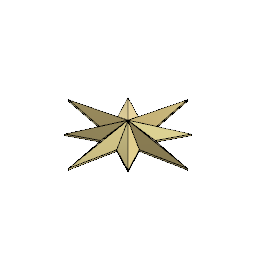
Star (Autodesk Fusion 360 design; units mm, degrees)
Autodesk Fusion 360 part; units mm, degrees
sketch "Outline" plane through (0, 0, 0) normal (0, 0, 1) x (1, 0, 0)
  line L0 (0, 0) -> (82.1329, 34.0206) construction
  line L1 (0, 0) -> (34.0206, 82.1329) construction
  line L2 (0, 0) -> (82.1329, -34.0206) construction
  line L3 (0, 0) -> (34.0206, -82.1329) construction
  line L4 (0, 0) -> (-82.1329, 34.0206) construction
  line L5 (0, 0) -> (-34.0206, -82.1329) construction
  line L6 (0, 0) -> (-82.1329, -34.0206) construction
  line L7 (0, 0) -> (-34.0206, 82.1329)
  line L8 (82.1329, 34.0206) -> (134.7038, 134.7038)
  line L9 (134.7038, 134.7038) -> (34.0206, 82.1329)
  line L10 (254, 0) -> (82.1329, 34.0206)
  line L11 (82.1329, -34.0206) -> (254, 0)
  line L12 (134.7038, -134.7038) -> (82.1329, -34.0206)
  line L13 (34.0206, -82.1329) -> (134.7038, -134.7038)
  line L14 (34.0206, 82.1329) -> (0, 254)
  line L15 (0, 254) -> (-34.0206, 82.1329)
  line L16 (-34.0206, 82.1329) -> (-134.7268, 134.6809)
  line L17 (-134.7268, 134.6809) -> (-82.1329, 34.0206)
  line L18 (-82.1329, 34.0206) -> (-254, 0)
  line L19 (-254, 0) -> (-82.1329, -34.0206)
  line L20 (-82.1329, -34.0206) -> (-134.7038, -134.7038)
  line L21 (-134.7038, -134.7038) -> (-34.0206, -82.1329)
  line L22 (-34.0206, -82.1329) -> (0, -254)
  line L23 (0, -254) -> (34.0206, -82.1329)
  line L24 (-134.7268, 134.6809) -> (0, 0) construction
  line L25 (0, 0) -> (134.7038, -134.7038) construction
  line L26 (0, 0) -> (0, 254) construction
  line L27 (0, 0) -> (134.7038, 134.7038) construction
  line L28 (0, 0) -> (0, -254) construction
  line L29 (-134.7038, -134.7038) -> (0, 0) construction
  line L30 (0, 0) -> (-254, 0) construction
  line L31 (0, 0) -> (254, 0) construction
  circle A0 centre (0, 0) radius 11.95 construction
  circle A1 centre (8.2884, 8.6084) radius 2.1
  circle A2 centre (-8.6084, 8.2884) radius 2.1
  circle A3 centre (-8.2884, -8.6084) radius 2.1
  circle A4 centre (8.6084, -8.2884) radius 2.1
  circle A5 centre (0, 0) radius 16.2
  line L32 (4.3489, 7.4725) -> (7.3024, 4.6287)
  line L33 (7.3024, 4.6287) -> (11.2419, 5.7647)
  line L34 (11.2419, 5.7647) -> (12.2279, 9.7444)
  line L35 (12.2279, 9.7444) -> (9.2744, 12.5881)
  line L36 (9.2744, 12.5881) -> (5.3349, 11.4521)
  line L37 (5.3349, 11.4521) -> (4.3489, 7.4725)
  line L38 (-7.4725, 4.3489) -> (-4.6287, 7.3024)
  line L39 (-4.6287, 7.3024) -> (-5.7647, 11.2419)
  line L40 (-5.7647, 11.2419) -> (-9.7444, 12.2279)
  line L41 (-9.7444, 12.2279) -> (-12.5881, 9.2744)
  line L42 (-12.5881, 9.2744) -> (-11.4521, 5.3349)
  line L43 (-11.4521, 5.3349) -> (-7.4725, 4.3489)
  line L44 (-11.2419, -5.7647) -> (-12.2279, -9.7444)
  line L45 (-12.2279, -9.7444) -> (-9.2744, -12.5881)
  line L46 (-9.2744, -12.5881) -> (-5.3349, -11.4521)
  line L47 (-5.3349, -11.4521) -> (-4.3489, -7.4725)
  line L48 (-4.3489, -7.4725) -> (-7.3024, -4.6287)
  line L49 (-7.3024, -4.6287) -> (-11.2419, -5.7647)
  line L50 (11.4521, -5.3349) -> (7.4725, -4.3489)
  line L51 (7.4725, -4.3489) -> (4.6287, -7.3024)
  line L52 (4.6287, -7.3024) -> (5.7647, -11.2419)
  line L53 (5.7647, -11.2419) -> (9.7444, -12.2279)
  line L54 (9.7444, -12.2279) -> (12.5881, -9.2744)
  line L55 (12.5881, -9.2744) -> (11.4521, -5.3349)
  line L56 (-82.1329, 34.0206) -> (-34.0206, 82.1329)
  line L57 (34.0206, 82.1329) -> (-34.0206, 82.1329)
  line L58 (34.0206, 82.1329) -> (82.1329, 34.0206)
  line L59 (82.1329, 34.0206) -> (82.1329, -34.0206)
  line L60 (82.1329, -34.0206) -> (34.0206, -82.1329)
  line L61 (34.0206, -82.1329) -> (-34.0206, -82.1329)
  line L62 (-34.0206, -82.1329) -> (-82.1329, -34.0206)
  line L63 (-82.1329, -34.0206) -> (-82.1329, 34.0206)
  line L64 (4.6287, -7.3024) -> (0, 0) construction
  line L65 (7.4725, -4.3489) -> (0, 0) construction
  line L66 (0, 0) -> (7.3024, 4.6287) construction
  line L67 (4.3489, 7.4725) -> (0, 0) construction
  circle A6 centre (0, 0) radius 25.4
  circle A7 centre (0, 0) radius 25.146
  circle A8 centre (0, 0) radius 4.1
  line L68 (-4.3489, -7.4725) -> (0, 0) construction
  line L69 (-7.3024, -4.6287) -> (0, 0) construction
  line L70 (-7.4725, 4.3489) -> (0, 0) construction
  line L71 (-4.6287, 7.3024) -> (0, 0) construction
  point P0 (8.2884, 8.6084)
  point P1 (-8.6084, 8.2884)
  point P2 (-8.2884, -8.6084)
  point P3 (8.6084, -8.2884)
  dimension "d21" = 254
  dimension "d22" = 190.5
  dimension "d23" = 88.9
  dimension "d24" = 45.01
  dimension "d25" = 22.5
  dimension "d26" = 22.5
  dimension "d27" = 22.5
  dimension "d28" = 22.5
  dimension "d29" = 22.5
  dimension "d30" = 22.5
  dimension "d31" = 22.5
  dimension "d32" = 22.5
  dimension "d33" = 45
  dimension "d73" = 23.9
  dimension "d74" = 4.2
  dimension "d79" = 360
  dimension "d80" = 32.4
  dimension "d90" = 4.1
  dimension "d91" = 4.1
  dimension "d92" = 4.1
  dimension "d93" = 4.1
  dimension "d151" = 50.8
  dimension "d155" = 50.292
  dimension "d167" = 8.2
  constraint coincident L0.start L1.start
  constraint perpendicular L25 L27
  constraint perpendicular L25 L29
  constraint vertical L26
  constraint horizontal L30
  constraint vertical L28
  constraint horizontal L31
  constraint equal L24 L29
  constraint equal L24 L27
  constraint equal L4 L7
  constraint equal L6 L7
  constraint equal L5 L7
  constraint equal L3 L7
  constraint equal L2 L7
  constraint equal L0 L7
  constraint equal L1 L7
  constraint coincident A0 P0
  constraint coincident P0 A1.centre
  constraint coincident P2 A3.centre
  constraint coincident P3 A4.centre
  constraint coincident P1 A2.centre
  constraint equal L64 L65
  constraint equal L66 L67
  constraint equal L70 L71
  constraint equal L68 L69
  measures "d21" distance of L0.start L14.end
  measures "d22" distance of L0.start L16.end
  measures "d23" distance of L7.end L0.start
  measures "d24" angle of L24 L26
  measures "d25" angle of L7 L26
  measures "d26" angle of L4 L30
  measures "d27" angle of L6 L30
  measures "d28" angle of L5 L28
  measures "d29" angle of L3 L28
  measures "d30" angle of L2 L31
  measures "d31" angle of L0 L31
  measures "d32" angle of L1 L26
  measures "d33" angle of L28 L29
  measures "d73" diameter of A0
  measures "d74" diameter of A1
  measures "d80" diameter of A5
  measures "d90" distance of L32.start P0
  measures "d91" distance of L38.start P1
  measures "d92" distance of L44.start P2
  measures "d93" distance of L50.start P3
  measures "d151" diameter of A6
  measures "d155" diameter of A7
  measures "d167" diameter of A8
extrude "Extrude1" add sketch "Outline" along normal blind 6.35 contours L8 L9 L58 | L56 L57 L58 L59 L60 L61 L62 L63 | L10 L11 L59 | L14 L15 L57 | L12 L13 L60 | L16 L17 L56 | L22 L23 L61 | L18 L19 L63 | L20 L21 L62 | A1 | A2 | A3 | A4 | A5 | L32 L33 L34 L35 L36 L37 | L38 L39 L40 L41 L42 L43 | L44 L45 L46 L47 L48 L49 | L50 L51 L52 L53 L54 L55 | A6 | A7 | A8 makes body 1
sketch "Profile" plane through (0, 0, 0) normal (1, 0, 0) x (0, 1, 0)
  line L0 (0, 57.15) -> (254, 6.35)
  line L1 (254, 6.35) -> (0, 6.35)
  line L2 (0, 0) -> (34.0206, 0)
  line L3 (82.1329, 0) -> (82.1329, 6.35) construction
  line L4 (82.1329, 6.35) -> (82.1329, 40.7234)
  line L5 (0, 6.35) -> (0, 57.15)
  point P0 (254, 6.35)
  point P1 (82.1329, 6.35)
  point P2 (82.1329, 0)
  dimension "d20" = 50.8
  constraint coincident P0 L0.end
  constraint coincident P2 L3.start
  constraint coincident L1 P1
  constraint perpendicular L1 L3
  constraint coincident P1 L3.end
  constraint coincident L0 L4.end
  constraint perpendicular L1 L4
  constraint perpendicular L1 L5
  measures "d20" distance of L1.end L0.start
loft "Loft1" add section 1 face at (139.4219, 0, 6.35) section 2 point at (0, 0, 57.15) on bodies 1 bodies 1
extrude "Extrude24" cut sketch "Outline" along normal blind 20.4 contours A1 | A2 | A3 | A4 | A5 | L32 L33 L34 L35 L36 L37 | L38 L39 L40 L41 L42 L43 | L44 L45 L46 L47 L48 L49 | L50 L51 L52 L53 L54 L55 | A6 | A7 | A8 bodies 1
extrude "Extrude30" add sketch "Outline" along normal blind 19.8 separate body contours A5 | L32 L33 L34 L35 L36 L37 | L38 L39 L40 L41 L42 L43 | L44 L45 L46 L47 L48 L49 | L50 L51 L52 L53 L54 L55 | A7 makes body 2
extrude "Extrude31" cut sketch "Outline" against normal blind 9 from surface at 20 contours L32 L33 L34 L35 L36 L37 | L38 L39 L40 L41 L42 L43 | L44 L45 L46 L47 L48 L49 | L50 L51 L52 L53 L54 L55 bodies 2
ref_plane "WorkPlane12" through (92.3995, -38.2731, 0) normal (0.382683, 0.92388, 0) x (-0.92388, 0.382683, 0)
ref_plane "WorkPlane13" through (38.2731, -92.3995, 0) normal (0.92388, 0.382683, 0) x (-0.382683, 0.92388, 0)
ref_plane "WorkPlane14" through (-38.2731, -92.3995, 0) normal (0.92388, -0.382683, 0) x (0.382683, 0.92388, 0)
split "Split15" by plane through (-38.2731, -92.3995, 0) normal (0.92388, -0.382683, 0) bodies 1 makes body 3 at (139.4219, 0, 0)
split "Split16" by plane through (38.2731, -92.3995, 0) normal (0.92388, 0.382683, 0) bodies 3 makes body 4 at (139.4219, 0, 0)
split "Split17" by plane through (92.3995, -38.2731, 0) normal (0.382683, 0.92388, 0) bodies 4 makes body 5 at (139.4219, 0, 0)
named bodies: "Star", "Long", "Short", "Two", "Core"
